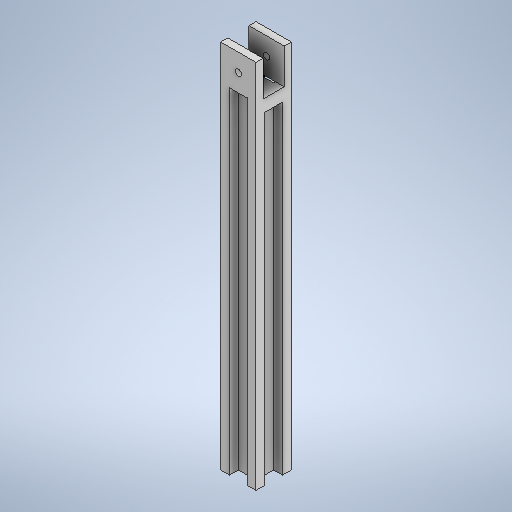
# Autodesk Inventor part: rail_principal
Saved by Autodesk Inventor 2025 (Build 290162000, 162)
## iProperties
Created: 2024-11-18
Part Number: rail_principal
Material: Générique
Document SubType Name: Modeling
Designer: chass
Density: 1 g/cm^3
Appearance: Par défaut
Author: chass
Autodesk Inventor part; units mm, degrees
ref_plane "YZ Plane" through (0, 0, 0) normal (1, 0, 0) x (0, 1, 0)
ref_plane "XZ Plane" through (0, 0, 0) normal (0, 1, 0) x (-1, 0, 0)
ref_plane "XY Plane" through (0, 0, 0) normal (0, 0, 1) x (1, 0, 0)
sketch "Esquisse1" plane through (0, 0, 0) normal (1, 0, 0) x (0, 1, 0)
  line L0 (95, 10) -> (-95, 10)
  line L1 (-95, 10) -> (-95, -10)
  line L2 (-95, -10) -> (95, -10)
  line L3 (95, -10) -> (95, 10)
  line L4 (95, 10) -> (-95, -10)
  line L5 (-95, 10) -> (95, -10)
  point P0 (0, 0)
  point P1 (0, 0)
  point P2 (0, 0)
  dimension "d0" = 190
  dimension "d1" = 20
  constraints: 12 end point, 2 midpoint, 2 parallel, 1 coincident, 1 horizontal, 1 perpendicular
  measures "d0" distance of L1.end L2.end
  measures "d1" distance of L2.end L0.start
extrude "Extrusion1" add sketch "Esquisse1" along normal blind 20
sketch "Esquisse2" plane through (0, 95, 10) normal (0, 1, 0) x (1, 0, 0)
  line L0 (20, 20) -> (20, 0) projected
  line L1 (0, 0) -> (20, 0)
  line L2 (20, 0) -> (20, 4)
  line L3 (20, 4) -> (0, 4)
  line L4 (0, 4) -> (0, 0)
  line L5 (0, 10) -> (20, 10)
  line L6 (0, 20) -> (20, 20)
  line L7 (20, 20) -> (20, 16)
  line L8 (20, 16) -> (0, 16)
  line L9 (0, 16) -> (0, 20)
  constraints: 18 end point, 5 symmetric about line, 2 parallel, 1 horizontal, 1 midpoint, 1 perpendicular, 1 point on line
extrude "Extrusion2" add sketch "Esquisse2" along normal blind 20
sketch "Esquisse3" plane through (0, -95, 10) normal (0, 0, 1) x (1, 0, 0)
  circle A0 centre (10, 200) radius 1.765
  line L0 (0, 0) -> (0, 210) projected
  line L1 (0, 210) -> (20, 210) projected
  point P0 (0, 95)
  dimension "d6" = 3.53
  dimension "d7" = 10
  dimension "d8" = 10
  constraints: 1 centre point
  measures "d6" diameter of A0
  measures "d7" distance from line of L0 A0.centre
  measures "d8" distance from line of L1 A0.centre
extrude "Extrusion3" cut sketch "Esquisse3" against normal blind 78.75
sketch "Esquisse4" plane through (0, -95, 10) normal (0, 0, 1) x (1, 0, 0)
  line L0 (20, 190) -> (0, 190) projected
  line L1 (5, 0) -> (15, 0)
  line L2 (15, 0) -> (15, 190)
  line L3 (15, 190) -> (5, 190)
  line L4 (5, 190) -> (5, 0)
  point P0 (0, 95)
  constraints: 8 end point, 2 parallel, 1 horizontal, 1 perpendicular, 1 point on line
extrude "Extrusion4" cut sketch "Esquisse4" against normal blind 5
sketch "Esquisse5" plane through (20, -95, -10) normal (0, 0, -1) x (-1, 0, 0)
  line L0 (5, 0) -> (0, 0) projected
  line L1 (15, 0) -> (15, 190) projected
  line L2 (5, 0) -> (15, 0)
  line L3 (15, 0) -> (15, 190)
  line L4 (15, 190) -> (5, 190)
  line L5 (5, 190) -> (5, 0)
  point P0 (20, 95)
  constraints: 8 end point, 2 parallel, 1 horizontal, 1 perpendicular
extrude "Extrusion5" cut sketch "Esquisse5" against normal blind 5
sketch "Esquisse6" plane through (20, 0, 0) normal (1, 0, 0) x (0, 0, -1)
  line L0 (-10, -95) -> (10, -95) projected
  line L1 (5, -95) -> (5, 95) projected
  line L2 (-5, -95) -> (5, -95)
  line L3 (5, -95) -> (5, 88)
  line L4 (5, 88) -> (-5, 88)
  line L5 (-5, 88) -> (-5, -95)
  point P0 (0, 0)
  constraints: 8 end point, 2 parallel, 2 point on line, 1 horizontal, 1 perpendicular
extrude "Extrusion6" cut sketch "Esquisse6" against normal blind 5
sketch "Esquisse7" plane through (0, 0, 0) normal (-1, 0, 0) x (0, 0, 1)
  line L0 (-5, 88) -> (-5, -95) projected
  line L1 (5, -95) -> (5, 95) projected
  line L2 (-5, -95) -> (5, -95)
  line L3 (5, -95) -> (5, 88)
  line L4 (5, 88) -> (-5, 88)
  line L5 (-5, 88) -> (-5, -95)
  point P0 (0, 0)
  constraints: 8 end point, 2 parallel, 1 horizontal, 1 perpendicular, 1 point on line
extrude "Extrusion7" cut sketch "Esquisse7" against normal blind 5
